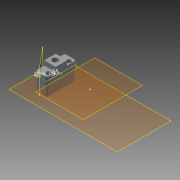
# Autodesk Inventor part: CAD:OPENSTOPBRKT
Saved by Autodesk Inventor 2015 (Build 190159000, 159)
## iProperties
Created: 2015-09-18
Material: Generic
Description: open endstop
Document SubType Name: Modeling
Designer: francis
Density: 1 g/cm^3
Appearance: Default
Part Category: insert part category here and press enter to fill value
Author: francis
Autodesk Inventor part; units mm, degrees
ref_plane "YZ Plane" through (0, 0, 0) normal (1, 0, 0) x (0, 1, 0)
ref_plane "XZ Plane" through (0, 0, 0) normal (0, 1, 0) x (-1, 0, 0)
ref_plane "Work Plane1" through (0, 0, 0) normal (0, 0, 1) x (1, 0, 0)
sketch "Sketch1" plane through (0, 0, 0) normal (0, 0, 1) x (1, 0, 0)
  circle A0 centre (-27.5, 9) radius 2 projected
  circle A1 centre (-27.5, -9) radius 2 projected
  circle A2 centre (-30.5, 0) radius 2.5 projected
  line L0 (-25, 13) -> (-25, -12.5061)
  line L1 (-35, -13) -> (-35, 13)
  line L2 (-25, -12.5061) -> (-25, -13)
  line L3 (-25, -13) -> (-35, -13)
  line L4 (-35, 13) -> (-25, 13)
  arc A3 (-2.9901, -1.4163) -> (-18.371, -4.3253) centre (-12.371, 6.067) ccw construction
  line L5 (-35, -13) -> (-35, 13) construction
  line L6 (-60.2, 0) -> (60.2, 0) construction
  point P0 (0, 0)
  dimension "d31" = 2.5
  dimension "d37" = 26
  constraints: 14 end point, 3 vertical, 2 horizontal, 2 point on circle, 1 centre point, 1 perpendicular, 3 other
  measures "d31" distance from line of L0 A0.centre
  measures "d37" distance of L1.start L1.end
ref_plane "Work Plane2" through (-37, -13, 19) normal (0, 0, -1) x (0, 1, 0)
extrude "Extrusion1" add sketch "Sketch1" along normal up to surface (19 mm away)
ref_plane "Work Plane3" through (-0.8627, 0, 12) normal (0, 0, 1) x (1, 0, 0)
sketch "Sketch4" plane through (-0.8627, 0, 12) normal (0, 0, 1) x (1, 0, 0)
  circle A0 centre (-29.6373, 0) radius 2.5 construction
  circle A1 centre (-26.6373, -9) radius 2 construction
  circle A2 centre (-26.6373, 9) radius 2 construction
  line L0 (-34.1373, -13) -> (-24.1373, -13) construction
  line L1 (-24.1373, -13) -> (-24.1373, 13) construction
  line L2 (-24.1373, 13) -> (-34.1373, 13) construction
  line L3 (-34.1373, 13) -> (-34.1373, -13) construction
  line L4 (-24.1373, 13) -> (-24.1373, -13) construction
  line L5 (-24.1373, -3.2174) -> (-34.1373, -11.6084) construction
  line L6 (-34.1373, -13) -> (-34.1373, 13) construction
  line L7 (-24.1373, -1.2593) -> (-34.1373, -9.6503) construction
  line L8 (-24.1373, 0.6988) -> (-34.1373, -7.6922) construction
  line L9 (-23.1842, -0.4595) -> (-35.6373, -10.9089)
  point P0 (0.8627, 0)
  dimension "d7" = 130
  dimension "d8" = 1.5
  dimension "d9" = 1.5
  dimension "d10" = 0.5
  dimension "d13" = 1.5
  constraints: 8 end point, 7 point on line, 2 parallel
  measures "d7" angle of L3 L5
  measures "d8" distance between parallel lines of L8 L7
  measures "d9" distance between parallel lines of L5 L7
  measures "d10" distance edge to line of A0 L8
  measures "d13" distance from line of L3 L9.end
ref_plane "Work Plane6" through (-35, -7.6922, 12) normal (-0.766, -0.6428, 0) x (0.6428, -0.766, 0)
sketch "Sketch7" plane through (-35, -7.6922, 12) normal (-0.766, -0.6428, 0) x (0.6428, -0.766, 0)
  point P0 (16.605, -12)
  point P1 (1.5, 0)
  point P2 (1.5, 0)
  point P3 (1.5, 0)
hole "Hole1" at (-34.0358, -8.8412, 12) direction (0.766, 0.6428, 0) diameter 2.459 end through all thread size "M3x0.5" class "6H" standard "ISO Metric profile"
hole "Hole2" at (-34.0358, -8.8412, 12) direction (-0.766, -0.6428, 0) diameter 2.459 end through all thread size "M3x0.5" class "6H" standard "ISO Metric profile"
sketch "Sketch9" plane through (-35, -13, 0) normal (-1, 0, 0) x (0, 0, 1)
  line L0 (19, 26) -> (15, 26)
  line L1 (15, 26) -> (15, 18)
  line L2 (15, 18) -> (19, 18)
  line L3 (19, 18) -> (19, 26)
  line L4 (19, 0) -> (15, 0)
  line L5 (15, 0) -> (15, 8)
  line L6 (15, 8) -> (19, 8)
  line L7 (19, 8) -> (19, 0)
  point P0 (0, 13)
  dimension "d32" = 4
  dimension "d33" = 8
  constraints: 16 end point, 4 parallel, 2 horizontal, 2 perpendicular, 1 collinear, 1 point on line
  measures "d32" distance of L1.end L2.end
  measures "d33" distance of L4.end L5.end
extrude "Extrusion2" cut sketch "Sketch9" against normal up to surface (10 mm away)
fillet "Fillet1" radius 2 4 edges at (-25, 13, 7.5) (-35, 13, 7.5) (-35, -13, 7.5) (-25, -13, 7.5)
body "Solid1"
